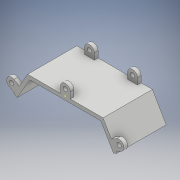
# Autodesk Inventor part: Capcture Zone2
Saved by Autodesk Inventor 2018 (Build 220112000, 112)
## iProperties
Created: 2017-10-13
Part Number: Capcture Zone2
Material: Generic
Document SubType Name: Modeling
Designer: BrisbaneMatt
Density: 1 g/cm^3
Appearance: Default
Author: BrisbaneMatt
Autodesk Inventor part; units mm, degrees
ref_plane "YZ Plane" through (0, 0, 0) normal (1, 0, 0) x (0, 1, 0)
ref_plane "XZ Plane" through (0, 0, 0) normal (0, 1, 0) x (-1, 0, 0)
ref_plane "XY Plane" through (0, 0, 0) normal (0, 0, 1) x (1, 0, 0)
sketch "Sketch1" plane through (0, 0, 0) normal (0, 1, 0) x (-1, 0, 0)
  line L0 (0, 0) -> (-30.6, 0)
  line L1 (0, 0) -> (30.6, 0)
  line L2 (30.6, 0) -> (41.764, -19.3366)
  line L3 (30.6, 0) -> (52.928, 0) construction
  line L4 (-30.6, 0) -> (-41.764, -19.3366)
  line L5 (-30.6, 0) -> (-8.272, 0) construction
  line L6 (0, 0) -> (0, 77)
  line L7 (0, 0) -> (0, -3)
  line L8 (-35.3569, -8.2392) -> (-32.7588, -9.7392)
  line L9 (35.0582, -7.7219) -> (32.4602, -9.2219)
  line L10 (32.4602, -9.2219) -> (28.8679, -3)
  line L11 (28.8679, -3) -> (0, -3)
  line L12 (0, -3) -> (-28.8679, -3)
  line L13 (-28.8679, -3) -> (-32.7588, -9.7392)
  line L14 (-32.7588, -9.7392) -> (-38.9714, -20.4998)
  line L15 (32.4602, -9.2219) -> (38.9714, -20.4998)
  arc A0 (38.9714, -20.4998) -> (41.764, -19.3366) centre (0, 77) ccw
  arc A1 (-41.764, -19.3366) -> (-38.9714, -20.4998) centre (0, 77) ccw
  dimension "d0" = 30.6
  dimension "d1" = 30.6
  dimension "d2" = 22.328
  dimension "d3" = 60
  dimension "d4" = 22.328
  dimension "d5" = 120
  dimension "d6" = 77
  dimension "d7" = 3
  dimension "d8" = 3
  dimension "d9" = 3
  constraints: 32 end point, 6 point on line, 5 horizontal, 4 perpendicular, 4 point on circle, 2 centre point, 2 equal length, 1 vertical
  measures "d0" distance of L0.start L0.end
  measures "d1" distance of L0.start L1.end
  measures "d2" distance of L1.end L2.end
  measures "d3" angle of L2 L3
  measures "d4" distance of L0.end L4.end
  measures "d5" angle of L4 L5
  measures "d6" distance of L0.start L6.end
  measures "d7" distance of L0.start L7.end
  measures "d8" distance of L8.start L8.end
  measures "d9" distance of L9.start L9.end
extrude "Extrusion1" add sketch "Sketch1" along normal blind 40
sketch "Sketch2" plane through (0, 0, 0) normal (0, -1, 0) x (1, 0, 0)
  line L0 (0, 0) -> (0, 5)
  circle A0 centre (0, 5) radius 1.5
  line L1 (-41.764, -19.3366) -> (-39.264, -15.0065)
  line L2 (-41.764, -19.3366) -> (-30.6, 0) projected
  line L3 (-39.264, -15.0065) -> (-43.5941, -12.5065)
  arc A1 (38.9714, -20.4998) -> (41.764, -19.3366) centre (0, 77) ccw projected
  line L4 (38.9714, -20.4998) -> (39.264, -15.0065)
  line L5 (30.6, 0) -> (41.764, -19.3366) projected
  line L6 (41.764, -19.3366) -> (39.264, -15.0065)
  line L7 (39.264, -15.0065) -> (43.5941, -12.5065)
  circle A2 centre (43.5941, -12.5065) radius 1.5
  circle A3 centre (-43.5941, -12.5065) radius 1.5
  circle A4 centre (-43.5941, -12.5065) radius 4
  circle A5 centre (0, 5) radius 4
  circle A6 centre (43.5941, -12.5065) radius 4
  line L8 (43.5941, -12.5065) -> (45.5941, -15.9706)
  line L9 (45.5941, -15.9706) -> (41.264, -18.4706)
  line L10 (43.5941, -12.5065) -> (41.5941, -9.0424)
  line L11 (41.5941, -9.0424) -> (37.264, -11.5424)
  line L12 (4, 5) -> (4, 0)
  line L13 (-30.6, 0) -> (30.6, 0) projected
  line L14 (-4, 5) -> (-4, 0)
  line L15 (-43.5941, -12.5065) -> (-45.5941, -15.9706)
  line L16 (-45.5941, -15.9706) -> (-41.264, -18.4706)
  line L17 (-41.764, -19.3366) -> (-30.6, 0) projected
  line L18 (-43.5941, -12.5065) -> (-41.5941, -9.0424)
  line L19 (-41.5941, -9.0424) -> (-37.264, -11.5424)
  dimension "d12" = 5
  dimension "d13" = 3
  dimension "d14" = 5
  dimension "d15" = 5
  dimension "d16" = 5.5011
  dimension "d17" = 5
  dimension "d18" = 3
  dimension "d19" = 8
  dimension "d20" = 8
  dimension "d21" = 8
  constraints: 32 end point, 9 point on line, 7 perpendicular, 6 centre point, 6 coincident, 6 point on circle, 4 tangent, 2 vertical, 1 collinear, 1 parallel
  measures "d12" distance of L0.start L0.end
  measures "d13" diameter of A0
  measures "d14" distance of L1.start L1.end
  measures "d15" distance of L1.end L3.end
  measures "d16" distance of L4.start L4.end
  measures "d17" distance of L4.end L7.end
  measures "d18" diameter of A2
  measures "d19" diameter of A4
  measures "d20" diameter of A5
  measures "d21" diameter of A6
extrude "Extrusion2" add sketch "Sketch2" against normal blind 3 contours L13 L14 A5 L0 | L0 A5 L12 L13 | A5 | L16 A4 L3 L1 | L3 A4 L19 L2 | L15 A3 L3 A4 | A4 L18 A3 L15 | L3 A3 L18 A4 | L15 L3 A3 | A3 L18 L15 | L3 L18 A3 | L7 A6 L9 L5 | L5 L11 A6 L7 | A6 L10 A2 L7 | L7 A2 L8 A6 | L8 A2 L10 A6 | A2 L10 L7 | L7 L8 A2 | L8 L10 A2
sketch "Sketch3" plane through (0, 3, 0) normal (0, 1, 0) x (1, 0, 0)
  arc A0 (41.5941, 9.0424) -> (45.5941, 15.9706) centre (43.5941, 12.5065) ccw projected
  circle A1 centre (43.5941, 12.5065) radius 1.5
  arc A2 (-45.5941, 15.9706) -> (-41.5941, 9.0424) centre (-43.5941, 12.5065) ccw projected
  circle A3 centre (-43.5941, 12.5065) radius 1.5
  point P0 (0, 0)
  dimension "d24" = 3
  constraints: 2 centre point, 2 coincident
  measures "d24" diameter of A1
extrude "Extrusion3" cut sketch "Sketch3" against normal blind 3
sketch "Sketch4" plane through (-30.6, 40, 0) normal (0, 0, 1) x (1, 0, 0)
  point P0 (30.6, -40)
sketch "Sketch5" plane through (0, 40, 0) normal (0, 1, 0) x (1, 0, 0)
  circle A0 centre (0, -5) radius 1.5 projected
  line L0 (0, -5) -> (17.465, -5)
  line L1 (0, -5) -> (-17.465, -5)
  circle A1 centre (-17.465, -5) radius 1.75
  circle A2 centre (17.465, -5) radius 1.75
  line L2 (-17.465, -5) -> (-21.465, -5)
  line L3 (-21.465, -5) -> (-21.465, 0)
  line L4 (-17.465, -5) -> (-13.465, -5)
  line L5 (-13.465, -5) -> (-13.465, 0)
  circle A3 centre (-17.465, -5) radius 4
  line L6 (17.465, -5) -> (13.465, -5)
  line L7 (13.465, -5) -> (13.465, 0)
  line L8 (-30.6, 0) -> (30.6, 0) projected
  line L9 (17.465, -5) -> (21.465, -5)
  line L10 (21.465, -5) -> (21.465, 0)
  circle A4 centre (17.465, -5) radius 4
  point P0 (0, 0)
  dimension "d27" = 17.465
  dimension "d28" = 17.465
  dimension "d29" = 3.5
  dimension "d30" = 4
  dimension "d31" = 4
  dimension "d32" = 4
  dimension "d33" = 4
  constraints: 20 end point, 5 point on line, 4 coincident, 4 perpendicular, 3 horizontal, 2 centre point, 2 horizontal alignment, 4 other
  measures "d27" distance of L0.start L0.end
  measures "d28" distance of L0.start L1.end
  measures "d29" diameter of A1
  measures "d30" distance of L2.start L2.end
  measures "d31" distance of L2.start L4.end
  measures "d32" distance of L6.start L6.end
  measures "d33" distance of L6.start L9.end
extrude "Extrusion4" add sketch "Sketch5" against normal blind 3 contours A4 L9 A2 L0 | L7 L8 L10 A4 | L0 A2 L9 A4 | A3 L2 A1 L1 | A3 L3 L8 L5 | L1 A1 L2 A3 | A2 L9 L0 | L1 L2 A1 picked at (18.233, -4.1331) picked at (-16.697, -4.1331)
sketch "Sketch6" plane through (0, 40, 0) normal (0, 1, 0) x (1, 0, 0)
  arc A0 (-19.215, -5) -> (-15.715, -5) centre (-17.465, -5) ccw projected
  line L0 (-19.215, -5) -> (-15.715, -5) projected
  circle A1 centre (-17.465, -5) radius 1.75
  arc A2 (15.715, -5) -> (19.215, -5) centre (17.465, -5) ccw projected
  line L1 (15.715, -5) -> (19.215, -5) projected
  circle A3 centre (17.465, -5) radius 1.75
  point P0 (0, 0)
  constraints: 2 coincident, 2 horizontal alignment, 4 other
extrude "Extrusion5" cut sketch "Sketch6" against normal blind 3 contours A1 L0 | A3 L1
sketch "Sketch7" plane through (0, 3, 0) normal (0, 1, 0) x (1, 0, 0)
  circle A0 centre (0, -5) radius 1.5 projected
  circle A1 centre (0, -5) radius 1.75
  circle A2 centre (43.5941, 12.5065) radius 1.5 projected
  circle A3 centre (43.5941, 12.5065) radius 1.75
  circle A4 centre (-43.5941, 12.5065) radius 1.5 projected
  circle A5 centre (-43.5941, 12.5065) radius 1.75
  point P0 (0, 0)
  dimension "d38" = 3.5
  dimension "d39" = 3.5
  dimension "d40" = 3.5
  constraints: 3 centre point, 3 coincident
  measures "d38" diameter of A1
  measures "d39" diameter of A3
  measures "d40" diameter of A5
extrude "Extrusion6" cut sketch "Sketch7" against normal blind 3 contours A1 | A3 | A4 | A5
body "Solid1"
